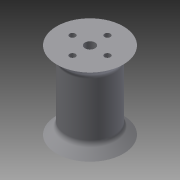
# Autodesk Inventor part: drum
Saved by Autodesk Inventor 2015 (Build 190159000, 159)
## iProperties
Created: 2015-03-06
Part Number: drum
Material: Generic
Document SubType Name: Modeling
Designer: jesse
Density: 1 g/cm^3
Appearance: Default
Author: jesse
Autodesk Inventor part; units mm, degrees
ref_plane "YZ Plane" through (0, 0, 0) normal (1, 0, 0) x (0, 1, 0)
ref_plane "XZ Plane" through (0, 0, 0) normal (0, 1, 0) x (-1, 0, 0)
ref_plane "XY Plane" through (0, 0, 0) normal (0, 0, 1) x (1, 0, 0)
sketch "Sketch2" plane through (0, 0, 0) normal (1, 0, 0) x (0, 1, 0)
  line L0 (0, 0) -> (0, -15.24)
  line L1 (0, -15.24) -> (-3.3101, -11.9299)
  line L2 (-5.5551, -11) -> (-29.8525, -11)
  line L3 (-32.0975, -11.9299) -> (-35.4076, -15.24)
  line L4 (-35.4076, -15.24) -> (-35.4076, 0)
  line L5 (-35.4076, 0) -> (0, 0)
  line L6 (-31.1676, -11) -> (-35.4076, -11) construction
  line L7 (-4.24, -11) -> (0, -11) construction
  arc A0 (-3.3101, -11.9299) -> (-5.5551, -11) centre (-5.5551, -14.175) ccw
  arc A1 (-29.8525, -11) -> (-32.0975, -11.9299) centre (-29.8525, -14.175) ccw
  dimension "d1" = 15.24
  dimension "d2" = 45
  dimension "d3" = 35.4076
  dimension "d5" = 3.175
  dimension "d6" = 11
  constraints: 16 end point, 7 point on line, 4 point on circle, 4 tangent, 2 centre point, 2 perpendicular, 2 vertical, 1 collinear, 1 equal radius, 1 horizontal, 1 parallel
  measures "d1" distance of L0.start L0.end
  measures "d2" angle of L0 L1
  measures "d3" distance of L4.end L0.start
  measures "d5" radius of A0
  measures "d6" distance between parallel lines of L5 L2
revolve "Revolution1" add sketch "Sketch2" angle 360 about axis through (0, -35.4076, 0) along (0, 1, 0)
sketch "Sketch3" plane through (0, 0, 0) normal (0, 1, 0) x (1, 0, 0)
  circle A0 centre (0, 0) radius 2.3241
  circle A1 centre (-8, 0) radius 1.3525
  circle A2 centre (0, 8) radius 1.3525
  circle A3 centre (8, 0) radius 1.3525
  circle A4 centre (0, -8) radius 1.3525
  point P0 (0, 0)
  point P1 (0, 0)
  dimension "d9" = 2.705
  dimension "d10" = 4.6482
  constraints: 5 centre point, 3 equal radius
  measures "d9" diameter of A1
  measures "d10" diameter of A0
extrude "Extrusion1" cut sketch "Sketch3" against normal through all
body "Solid1"
